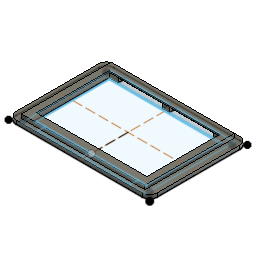
Zeiss_Plate_IonOptix-insert v1 (Autodesk Fusion 360 design; units mm, degrees)
Autodesk Fusion 360 part; units mm, degrees
sketch "Sketch1" plane through (0, 0, 0) normal (0, 1, 0) x (1, 0, 0)
  line L0 (-8.5, 0) -> (-150.5, 0)
  line L1 (-159, 8.5) -> (-159, 101.5)
  line L2 (-150.5, 110) -> (-8.5, 110)
  line L3 (0, 101.5) -> (0, 8.5)
  line L4 (0, 55) -> (-159, 55) construction
  line L5 (-79.5, 0) -> (-79.5, 110) construction
  line L6 (-10, 4.5) -> (-149, 4.5)
  line L7 (-149, 4.5) -> (-149, 105.5)
  line L8 (-149, 105.5) -> (-10, 105.5)
  line L9 (-10, 105.5) -> (-10, 4.5)
  line L10 (-79.5, 14) -> (-17.25, 14) construction
  line L11 (-17.25, 14) -> (-141.75, 14)
  line L12 (-141.75, 14) -> (-141.75, 96)
  line L13 (-141.75, 96) -> (-17.25, 96)
  line L14 (-17.25, 96) -> (-17.25, 14)
  line L15 (-79.5, 55) -> (-79.5, 12.25) construction
  line L16 (-79.5, 12.25) -> (-15.625, 12.25) construction
  line L17 (-15.625, 12.25) -> (-143.375, 12.25)
  line L18 (-143.375, 12.25) -> (-143.375, 97.75)
  line L19 (-143.375, 97.75) -> (-15.625, 97.75)
  line L20 (-15.625, 97.75) -> (-15.625, 12.25)
  arc A0 (-8.5, 0) -> (0, 8.5) centre (-8.5, 8.5) ccw
  arc A1 (0, 101.5) -> (-8.5, 110) centre (-8.5, 101.5) ccw
  arc A2 (-150.5, 110) -> (-159, 101.5) centre (-150.5, 101.5) ccw
  arc A3 (-159, 8.5) -> (-150.5, 0) centre (-150.5, 8.5) ccw
  line L21 (-143.375, 97.75) -> (-133.375, 97.75) construction
  line L22 (-133.375, 97.75) -> (-83.375, 97.75) construction
  line L23 (-83.375, 97.75) -> (-83.375, 105.75)
  line L24 (-83.375, 105.75) -> (-133.375, 105.75)
  line L25 (-133.375, 105.75) -> (-133.375, 97.75)
  line L26 (-15.625, 97.75) -> (-25.625, 97.75) construction
  line L27 (-25.625, 97.75) -> (-75.625, 97.75) construction
  line L28 (-75.625, 97.75) -> (-75.625, 105.75)
  line L29 (-75.625, 105.75) -> (-25.625, 105.75)
  line L30 (-25.625, 105.75) -> (-25.625, 97.75)
  line L31 (-141.75, 14) -> (-131.75, 14)
  line L32 (-131.75, 14) -> (-81.75, 14)
  line L33 (-81.75, 14) -> (-81.75, 6)
  line L34 (-81.75, 6) -> (-131.75, 6)
  line L35 (-131.75, 6) -> (-131.75, 14)
  line L36 (-17.25, 14) -> (-27.25, 14)
  line L37 (-27.25, 14) -> (-77.25, 14)
  line L38 (-77.25, 14) -> (-77.25, 6)
  line L39 (-77.25, 6) -> (-27.25, 6)
  line L40 (-27.25, 6) -> (-27.25, 14)
  point P0 (-159, 0)
  point P1 (0, 110)
  dimension "d1" = 159
  dimension "d2" = 110
  dimension "d5" = 139
  dimension "d6" = 101
  dimension "d9" = 124.5
  dimension "d10" = 82
  dimension "d11" = 42.75
  dimension "d12" = 63.875
  dimension "d13" = 127.75
  dimension "d14" = 85.5
  dimension "d15" = 8.5
  dimension "d16" = 8.5
  dimension "d19" = 8.5
  dimension "d20" = 8.5
  dimension "d31" = 10
  dimension "d32" = 50
  dimension "d33" = 8
  dimension "d34" = 10
  dimension "d35" = 50
  dimension "d36" = 8
  dimension "d43" = 10
  dimension "d44" = 50
  dimension "d45" = 8
  dimension "d46" = 10
  dimension "d47" = 50
  dimension "d48" = 8
  constraint horizontal L0
  constraint vertical L1
  constraint horizontal L2
  constraint vertical L3
  constraint horizontal L6
  constraint vertical L7
  constraint horizontal L8
  constraint vertical L9
  constraint perpendicular L5 L10
  constraint horizontal L11
  constraint vertical L12
  constraint horizontal L13
  constraint vertical L14
  constraint midpoint L4 L15.start
  constraint perpendicular L11 L15
  constraint perpendicular L15 L16
  constraint horizontal L17
  constraint vertical L18
  constraint horizontal L19
  constraint vertical L20
  constraint coincident L0 L5.start
  constraint coincident L3 L4.start
  constraint coincident origin L0
  constraint coincident origin L3
  constraint tangent L0 A0
  constraint tangent L3 A0
  constraint coincident L2 L5.end
  constraint coincident P1 L2
  constraint coincident P1 L3
  constraint tangent L2 A1
  constraint tangent L3 A1
  constraint coincident L1 L4.end
  constraint tangent L1 A2
  constraint tangent L2 A2
  constraint coincident P0 L0
  constraint coincident P0 L1
  constraint tangent L0 A3
  constraint tangent L1 A3
  constraint perpendicular L18 L21
  constraint horizontal L22
  constraint vertical L23
  constraint horizontal L24
  constraint vertical L25
  constraint perpendicular L20 L26
  constraint horizontal L27
  constraint vertical L28
  constraint horizontal L29
  constraint vertical L30
  constraint perpendicular L12 L31
  constraint horizontal L32
  constraint vertical L33
  constraint horizontal L34
  constraint vertical L35
  constraint perpendicular L14 L36
  constraint horizontal L37
  constraint vertical L38
  constraint horizontal L39
  constraint vertical L40
  measures "d1" distance of origin P0
  measures "d2" distance of origin P1
  measures "d5" distance of L6.start L6.end
  measures "d6" distance of L6.start L8.end
  measures "d9" distance of L10.end L11.end
  measures "d10" distance of L10.end L13.end
  measures "d11" distance of L15.start L15.end
  measures "d12" distance of L15.end L16.end
  measures "d13" distance of L16.end L17.end
  measures "d14" distance of L16.end L19.end
  measures "d15" radius of A0
  measures "d16" radius of A1
  measures "d19" radius of A2
  measures "d20" radius of A3
  measures "d31" distance of L18.end L21.end
  measures "d32" distance of L21.end L22.end
  measures "d33" distance of L21.end L24.end
  measures "d34" distance of L19.end L26.end
  measures "d35" distance of L26.end L27.end
  measures "d36" distance of L26.end L29.end
  measures "d43" distance of L11.end L31.end
  measures "d44" distance of L31.end L32.end
  measures "d45" distance of L31.end L34.end
  measures "d46" distance of L10.end L36.end
  measures "d47" distance of L36.end L37.end
  measures "d48" distance of L36.end L39.end
extrude "Extrude1" add sketch "Sketch1" along normal blind 1 contours L0 L1 L2 L3 A0 A1 A2 A3 | L8 L28 L29 L30 | L8 L23 L24 L25
extrude "Extrude2" cut 1 faces at (-152.3333, 1, -70.5) along direction (0, -1, 0) blind 1
extrude "Extrude3" add sketch "Sketch1" along normal blind 4 contours L0 L1 L2 L3 A0 A1 A2 A3 | L8 L28 L29 L30 | L8 L23 L24 L25
extrude "Extrude4" add sketch "Sketch1" along normal blind 8.5 contours L6 L7 L8 L9 L17 L18 L19 L20 L25 L30 L33 L34 L35 L38 L39 L40 | L8 L19 L28 L30 | L8 L19 L23 L25 | L8 L19 L23 L28 | L17 L38 L39 L40 | L17 L33 L34 L35
extrude "Extrude5" add sketch "Sketch1" along normal blind 8.5 contours L11 L12 L13 L14 L17 L18 L19 L20 L31 L35 L36 L40 | L11 L17 L37 L38 L40 | L11 L17 L32 L33 L35 | L11 L17 L33 L38
extrude "Extrude6" cut sketch "Sketch1" along normal blind 7 contours L11 L12 L13 L14 L17 L18 L19 L20 L31 L35 L36 L40 | L11 L17 L37 L38 L40 | L11 L17 L32 L33 L35 | L11 L17 L33 L38
extrude "Extrude8" cut sketch "Sketch1" along normal blind 5 contours L8 L19 L28 L30
extrude "Extrude9" cut sketch "Sketch1" along normal blind 5 contours L8 L19 L23 L25
extrude "Extrude10" cut sketch "Sketch1" along normal blind 5 contours L17 L33 L34 L35
extrude "Extrude11" cut sketch "Sketch1" along normal blind 5 contours L17 L38 L39 L40
extrude "Extrude7" [suppressed]
